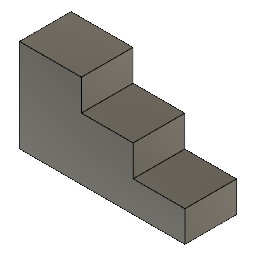
Tut1_P1(extrude command) (Autodesk Fusion 360 design; units mm, degrees)
Autodesk Fusion 360 part; units mm, degrees
sketch "Sketch1" plane through (0, 0, 0) normal (0, 1, 0) x (1, 0, 0)
  line L0 (0, 0) -> (0, -57.15)
  line L1 (0, 0) -> (101.6, 0)
  line L2 (0, -57.15) -> (38.1, -57.15)
  line L3 (38.1, -57.15) -> (38.1, -38.1)
  line L4 (38.1, -38.1) -> (69.85, -38.1)
  line L5 (69.85, -38.1) -> (69.85, -19.05)
  line L6 (69.85, -19.05) -> (101.6, -19.05)
  line L7 (101.6, -19.05) -> (101.6, 0)
  dimension "d2" = 57.15
  dimension "d3" = 101.6
  dimension "d4" = 38.1
  dimension "d5" = 19.05
  dimension "d6" = 31.75
  dimension "d7" = 19.05
  measures "d7" distance of L0.start
extrude "Extrude1" add sketch "Sketch1" along normal mid plane 31.75
equation "d8 = ( 1.25 / 2 ) * 1 in"
